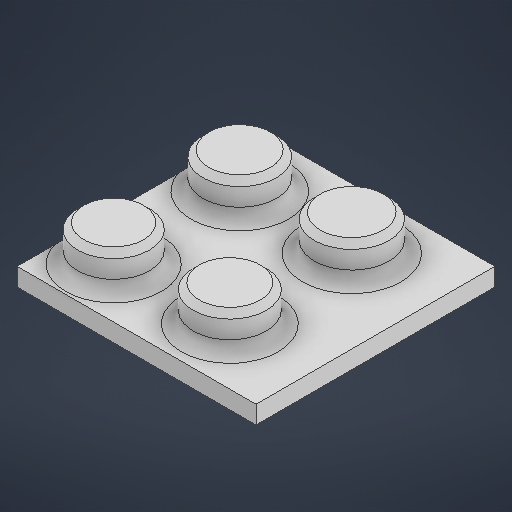
# Autodesk Inventor part: heligearPressFitTester
Saved by Autodesk Inventor 2026.1 (Build 301233020, 233B)
## iProperties
Created: 2026-02-13
Part Number: heligearPressFitTester
Material: Generic
Document SubType Name: Modeling
Designer: Dylan
Density: 1 g/cm^3
Appearance: Default
Author: Dylan
Autodesk Inventor part; units mm, degrees
ref_plane "YZ Plane" through (0, 0, 0) normal (1, 0, 0) x (0, 1, 0)
ref_plane "XZ Plane" through (0, 0, 0) normal (0, 1, 0) x (-1, 0, 0)
ref_plane "XY Plane" through (0, 0, 0) normal (0, 0, 1) x (1, 0, 0)
sketch "Sketch2" plane through (0, 0, 0) normal (0, 1, 0) x (-1, 0, 0)
  line L0 (0, 0) -> (-20, 0)
  line L1 (-20, 0) -> (-20, -20)
  line L2 (-20, -20) -> (0, -20)
  line L3 (0, -20) -> (0, 0)
  dimension "d0" = 20
  dimension "d1" = 20
  constraints: 8 end point, 2 parallel, 1 horizontal, 1 perpendicular
  measures "d0" distance of L2.end L1.end
  measures "d1" distance of L1.end L0.end
extrude "Extrusion1" add sketch "Sketch2" along normal blind 1.5
sketch "Sketch3" plane through (0, 1.5, 0) normal (0, 1, 0) x (1, 0, 0)
  circle A0 centre (3.8617, 4.2192) radius 3
  circle A1 centre (13.0724, 4.7341) radius 3.05
  circle A2 centre (3.8617, 14.7744) radius 3.075
  circle A3 centre (13.0724, 14.946) radius 3.125
  point P0 (0, 0)
  dimension "d4" = 6
  dimension "d5" = 6.1
  dimension "d6" = 6.15
  dimension "d7" = 6.25
  constraints: 4 centre point
  measures "d4" diameter of A0
  measures "d5" diameter of A1
  measures "d6" diameter of A2
  measures "d7" diameter of A3
extrude "Extrusion2" add sketch "Sketch3" along normal blind 3
fillet "Fillet1" radius 1 4 edges at (10.0224, 1.5, -4.7341) (0.8617, 1.5, -4.2192) (0.7867, 1.5, -14.7744) (9.9474, 1.5, -14.946)
chamfer "Chamfer1" distance 0.5 angle 45 4 edges at (10.0224, 4.5, -4.7341) (9.9474, 4.5, -14.946) (0.7867, 4.5, -14.7744) (0.8617, 4.5, -4.2192)
body "Solid1"
